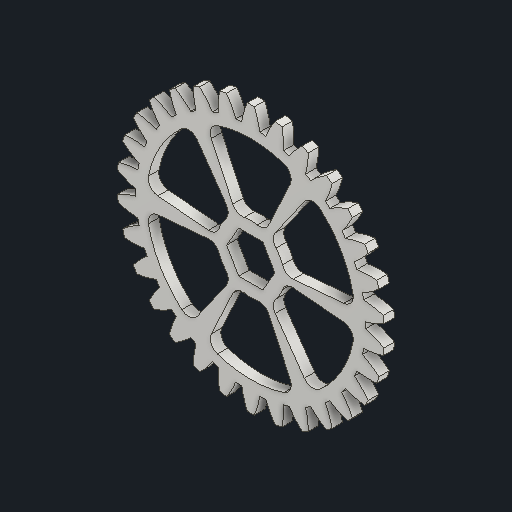
# Autodesk Inventor part: Spur Gear2
Saved by Autodesk Inventor 2026.2 (Build 302298010, 298A)
## iProperties
CustomPartVersion: 1
Created: 2026-04-01
Part Number: Spur Gear2
Material: Steel
Document SubType Name: Modeling
Designer: 4aida
Categories: <?xml version="1.0" encoding="UTF-16"?> <MemberInstance><Categories><FamilyTemplate><FamilyTemplateParameter ValueType="xs:double" Id="1" ObjectReferenceKey="da_z" ObjectType="kUserParameterObject"/><FamilyTemplateParameter ValueType="xs:double" Id="2" ObjectReferenceKey="da_b" ObjectType="kUserParameterObject"/><FamilyTemplateParameter ValueType="xs:double" Id="3" ObjectReferenceKey="da_beta" ObjectType="kUserParameterObject"/><FamilyTemplateParameter ValueType="xs:double" Id="4" ObjectReferenceKey="da_da" ObjectType="kUserParameterObject"/><FamilyTemplateParameter ValueType="xs:double" Id="5" ObjectReferenceKey="da_aw" ObjectType="kUserParameterObject"/><FamilyTemplateParameter ValueType="xs:string" Id="6" ObjectReferenceKey="EAIAABAAAAC/AAAAAAAAAIAAAAAAAAAA" ObjectType="83910656" SubObjectId="SurfaceGeometry"/></FamilyTemplate><ParamToTemplateMap><ParamToTemplate CategoryParameter="//CategoryParameter[@InternalName='046C89C9-8512-4d59-83FE-43B91F4F132A']" TemplateParameter="1"/><ParamToTemplate CategoryParameter="//CategoryParameter[@InternalName='2552DF32-E462-4b46-AEBF-C6C7768E72AC']" TemplateParameter="2"/><ParamToTemplate CategoryParameter="//CategoryParameter[@InternalName='C9EE641D-15FC-4fae-A226-E94C4372FDD7']" TemplateParameter="3"/><ParamToTemplate><ParamToTemplate CategoryParameter="//CategoryParameter[@InternalName='00B6519A-459B-49c7-AD84-2E56D39A5744']" ConstantValue="0.000000"/></ParamToTemplate><ParamToTemplate><ParamToTemplate CategoryParameter="//CategoryParameter[@InternalName='04B31F0E-C7A6-4894-AA32-9629BEFACF47']" ConstantValue="1.000000"/></ParamToTemplate><ParamToTemplate><ParamToTemplate CategoryParameter="//CategoryParameter[@InternalName='43CBEC2E-7847-49e7-A936-2F7889FCB2D9']" ConstantValue="0.250000"/></ParamToTemplate><ParamToTemplate><ParamToTemplate CategoryParameter="//CategoryParameter[@InternalName='B1EFC894-105D-4ebd-86BF-FA20ED196853']" ConstantValue="0.350000"/></ParamToTemplate><ParamToTemplate><ParamToTemplate CategoryParameter="//CategoryParameter[@InternalName='51175063-3D10-4879-93E8-6246FE8B403D']" ConstantValue="2061532430.657340"/></ParamToTemplate><ParamToTemplate><ParamToTemplate CategoryParameter="//CategoryParameter[@InternalName='A3A52E27-4454-46a9-B0BD-C932399B70AF']" ConstantValue="0.300000"/></ParamToTemplate><ParamToTemplate><ParamToTemplate CategoryParameter="//CategoryParameter[@InternalName='91B76062-C214-41d9-B1B9-14D2AB99603D']" ConstantValue="0.254000"/></ParamToTemplate><ParamToTemplate><ParamToTemplate CategoryParameter="//CategoryParameter[@InternalName='374E806E-8B8A-4dda-A9AA-1039D6500AD2']" ConstantValue="3.937008"/></ParamToTemplate><ParamToTemplate><ParamToTemplate CategoryParameter="//CategoryParameter[@InternalName='2D373A89-B862-43d6-8D0B-0CBF12AB9F6C']" ConstantValue="0.349066"/></ParamToTemplate><ParamToTemplate CategoryParameter="//CategoryParameter[@InternalName='37777632-D6A2-4fac-9D53-DB8ACD95C989']" TemplateParameter="4"/><ParamToTemplate CategoryParameter="//CategoryParameter[@InternalName='FD1017F1-B727-4f7e-9707-0F86F1FF9423']" TemplateParameter="5"/><ParamToTemplate><ParamToTemplate CategoryParameter="//CategoryParameter[@InternalName='9E1B4470-B2D3-4ff1-B813-535BB4CDF51A']" ConstantValue="3523220.976809"/></ParamToTemplate><ParamToTemplate><ParamToTemplate CategoryParameter="//CategoryParameter[@InternalName='F8452263-BFF6-458c-9FB1-07C4B99E95CD']" ConstantValue="11397033.805607"/></ParamToTemplate><ParamToTemplate><ParamToTemplate CategoryParameter="//CategoryParameter[@InternalName='3E3BB259-FD49-497f-8171-6EBC954A3479']" ConstantValue="2.000000"/></ParamToTemplate><ParamToTemplate CategoryParameter="//CategoryParameter[@InternalName='27C3BAF2-7550-4e4b-AE2C-0DB134B7D9B7']" TemplateParameter="6"/></ParamToTemplateMap><Category DisplayName="Gear" InternalName="DC85795E-93AB-48d5-8EEE-5A27447B64BD" Mnemonic="Gear"><CategoryParameter DisplayName="z" InternalName="046C89C9-8512-4d59-83FE-43B91F4F132A" Mnemonic="z"/><CategoryParameter DisplayName="b" InternalName="2552DF32-E462-4b46-AEBF-C6C7768E72AC" Mnemonic="b"/><CategoryParameter DisplayName="||b|" InternalName="C9EE641D-15FC-4fae-A226-E94C4372FDD7" Mnemonic="beta"/><CategoryParameter DisplayName="x" InternalName="00B6519A-459B-49c7-AD84-2E56D39A5744" Mnemonic="x"/><CategoryParameter DisplayName="a*" InternalName="04B31F0E-C7A6-4894-AA32-9629BEFACF47" Mnemonic="a"/><CategoryParameter DisplayName="c*" InternalName="43CBEC2E-7847-49e7-A936-2F7889FCB2D9" Mnemonic="c"/><CategoryParameter DisplayName="r|.f|*" InternalName="B1EFC894-105D-4ebd-86BF-FA20ED196853" Mnemonic="rf"/><CategoryParameter DisplayName="E" InternalName="51175063-3D10-4879-93E8-6246FE8B403D" Mnemonic="E"/><CategoryParameter DisplayName="||m|" InternalName="A3A52E27-4454-46a9-B0BD-C932399B70AF" Mnemonic="mi"/><Category DisplayName="SpurGear" InternalName="26C5A22E-A91E-4dfd-A3B3-23CCAFAE1764" Mnemonic="SpurGear"><CategoryParameter DisplayName="m" InternalName="91B76062-C214-41d9-B1B9-14D2AB99603D" Mnemonic="m"/><CategoryParameter DisplayName="P" InternalName="374E806E-8B8A-4dda-A9AA-1039D6500AD2" Mnemonic="PP"/><CategoryParameter DisplayName="||a|" InternalName="2D373A89-B862-43d6-8D0B-0CBF12AB9F6C" Mnemonic="alpha"/><CategoryParameter DisplayName="d|.a|" InternalName="37777632-D6A2-4fac-9D53-DB8ACD95C989" Mnemonic="da"/><CategoryParameter DisplayName="a|.w|" InternalName="FD1017F1-B727-4f7e-9707-0F86F1FF9423" Mnemonic="aw"/><CategoryParameter DisplayName="||s||.Flim|" InternalName="9E1B4470-B2D3-4ff1-B813-535BB4CDF51A" Mnemonic="sFlim"/><CategoryParameter DisplayName="||s||.Hlim|" InternalName="F8452263-BFF6-458c-9FB1-07C4B99E95CD" Mnemonic="sHlim"/><CategoryParameter DisplayName="type" InternalName="3E3BB259-FD49-497f-8171-6EBC954A3479" Mnemonic="type"/><CategoryParameter DisplayName="PitchDiameter" InternalName="27C3BAF2-7550-4e4b-AE2C-0DB134B7D9B7" Mnemonic="IDS_PITCHDIAM"/></Category></Category></Categories></MemberInstance>
Density: 1 g/cm^3
Appearance: Steel
Author: 4aida
Autodesk Inventor part; units mm, degrees
ref_plane "YZ Plane" through (0, 0, 0) normal (1, 0, 0) x (0, 1, 0)
ref_plane "XZ Plane" through (0, 0, 0) normal (0, 1, 0) x (-1, 0, 0)
ref_plane "XY Plane" through (0, 0, 0) normal (0, 0, 1) x (1, 0, 0)
sketch "Sketch1" plane through (0, 0, 0) normal (0, 0, 1) x (1, 0, 0)
  circle A0 centre (0, 0) radius 40.64
  dimension "d0" = 81.28
  constraints: 1 centre point
  measures "d0" diameter of A0
extrude "Extrusion1" add sketch "Sketch1" along normal blind 3.175
sketch "Sketch2" plane through (0, 0, 0) normal (0, 0, -1) x (-1, 0, 0)
  circle A0 centre (0, 0) radius 40.64 projected
  circle A1 centre (0, 0) radius 38.1
  dimension "d3" = 76.2
  constraints: 1 centre point, 1 coincident
  measures "d3" diameter of A1
surface extrude "Pitch Diameter" sketch "Sketch2" against normal through all shown no curves A1
ref_plane "Work Plane1" through (0, 0, 0) normal (1, 0, 0) x (0, 1, 0)
ref_plane "Work Plane2" through (0, 0, 0) normal (0.9945219, 0.1045285, 0) x (0, 0, 1)
ref_plane "Work Plane3" through (0, 0, 1.5875) normal (0, 0, -1) x (-1, 0, 0)
spur gear teeth "Spur Gear" teeth 30 pitch diameter 76.2 tip diameter 81.28 root diameter 69.85 face width 3.175 start plane through (0, 0, 0) normal (0, 0, -1) x (-1, 0, 0)
sketch "Sketch3" plane through (0, 0, 3.175) normal (0, 0, 1) x (1, 0, 0)
  line L0 (3.6662, 6.35) -> (7.3323, 0)
  line L1 (7.3323, 0) -> (3.6662, -6.35)
  line L2 (3.6662, -6.35) -> (-3.6662, -6.35)
  line L3 (-3.6662, -6.35) -> (-7.3323, 0)
  line L4 (-7.3323, 0) -> (-3.6662, 6.35)
  line L5 (-3.6662, 6.35) -> (3.6662, 6.35)
  circle A0 centre (0, 0) radius 10.16
  circle A1 centre (0, 0) radius 31.75
  line L6 (31.6292, 2.7672) -> (10.1213, 0.8855)
  line L7 (10.1213, -0.8855) -> (31.6292, -2.7672)
  line L8 (0, 0) -> (31.75, 0) construction
  line L9 (13.4181, 28.7753) -> (4.2938, 9.2081)
  line L10 (5.8275, 8.3226) -> (18.2111, 26.0081)
  line L11 (0, 0) -> (15.875, 27.4963) construction
  line L12 (-18.2111, 26.0081) -> (-5.8275, 8.3226)
  line L13 (-4.2938, 9.2081) -> (-13.4181, 28.7753)
  line L14 (0, 0) -> (-15.875, 27.4963) construction
  line L15 (-31.6292, -2.7672) -> (-10.1213, -0.8855)
  line L16 (-10.1213, 0.8855) -> (-31.6292, 2.7672)
  line L17 (0, 0) -> (-31.75, 0) construction
  line L18 (-13.4181, -28.7753) -> (-4.2938, -9.2081)
  line L19 (-5.8275, -8.3226) -> (-18.2111, -26.0081)
  line L20 (0, 0) -> (-15.875, -27.4963) construction
  line L21 (18.2111, -26.0081) -> (5.8275, -8.3226)
  line L22 (4.2938, -9.2081) -> (13.4181, -28.7753)
  line L23 (0, 0) -> (15.875, -27.4963) construction
  point P0 (3.6662, 6.35)
  point P1 (-3.6662, 6.35)
  point P2 (-7.3323, 0)
  point P3 (-3.6662, -6.35)
  point P4 (3.6662, -6.35)
  point P5 (-31.6292, 2.7672)
  point P6 (-10.1213, 0.8855)
  point P7 (-5.8275, 8.3226)
  point P8 (-18.2111, 26.0081)
  point P9 (-18.2111, -26.0081)
  point P10 (-5.8275, -8.3226)
  point P11 (-10.1213, -0.8855)
  point P12 (-31.6292, -2.7672)
  point P13 (13.4181, -28.7753)
  point P14 (4.2938, -9.2081)
  point P15 (-4.2938, -9.2081)
  point P16 (-13.4181, -28.7753)
  point P17 (5.8275, 8.3226)
  point P18 (5.8275, -8.3226)
  point P19 (18.2111, -26.0081)
  point P20 (-13.4181, 28.7753)
  point P21 (-4.2938, 9.2081)
  point P22 (13.4181, 28.7753)
  dimension "d20" = 10
  dimension "d21" = 5
  dimension "d22" = 12.7
  dimension "d23" = 20.32
  dimension "d24" = 63.5
  dimension "d27" = 360
  constraints: 48 end point, 18 point on line, 5 coincident, 5 point on circle, 2 centre point, 1 horizontal, 78 other
  measures "d20" angle of L7 L6
  measures "d21" angle of L7 L8
  measures "d22" distance between parallel lines of L2 L5
  measures "d23" diameter of A0
  measures "d24" diameter of A1
extrude "Extrusion2" cut sketch "Sketch3" against normal through all contours L0 L1 L2 L3 L4 L5 | A0 L10 A1 L6 | L7 A1 L21 A0 | A0 L13 A1 L9 | L22 A1 L18 A0 | A0 L16 A1 L12 | L19 A1 L15 A0
fillet "Fillet1" radius 3.175 24 edges at (-5.8275, -8.3226, 1.5875) (-4.2938, -9.2081, 1.5875) (-10.1213, -0.8855, 1.5875) (-10.1213, 0.8855, 1.5875) (-5.8275, 8.3226, 1.5875) (-4.2938, 9.2081, 1.5875) (4.2938, 9.2081, 1.5875) (5.8275, 8.3226, 1.5875) (10.1213, 0.8855, 1.5875) (10.1213, -0.8855, 1.5875) (4.2938, -9.2081, 1.5875) (5.8275, -8.3226, 1.5875) (18.2111, -26.0081, 1.5875) (13.4181, -28.7753, 1.5875) (-13.4181, -28.7753, 1.5875) (-18.2111, -26.0081, 1.5875) (-31.6292, -2.7672, 1.5875) (-31.6292, 2.7672, 1.5875) (-18.2111, 26.0081, 1.5875) (-13.4181, 28.7753, 1.5875) (13.4181, 28.7753, 1.5875) (18.2111, 26.0081, 1.5875) (31.6292, 2.7672, 1.5875) (31.6292, -2.7672, 1.5875)
equation "\"d0\" = da_da"
equation "\"d1\" = da_b"
equation "\"d21\" = 0.5 * d20"
equation "\"d3\" = da_d"
equation "\"d15\" = da_aw"
equation "\"d19\" = da_aw"
equation "\"da_da\" = 81.28"
equation "\"da_b\" = 3.175"
equation "\"da_d\" = 76.2"
equation "\"da_aw\" = 50.8"
body "Solid1"
body "Srf1"
